Autodesk Inventor part; units mm, degrees
(part 2 of 2)
  arc A565 (31.0706, -18.1829) -> (31.0657, -18.0745) centre (30.9843, -18.1324) ccw
  arc A566 (31.0657, -18.0745) -> (30.4409, -17.2728) centre (21.5601, -24.8386) ccw
  arc A567 (30.4409, -17.2728) -> (30.3559, -17.1866) centre (29.8098, -17.8105) ccw
  arc A568 (29.7735, -16.6368) -> (30.3559, -17.1866) centre (37.4523, -9.0861) ccw
  arc A569 (29.6902, -16.0485) -> (29.7735, -16.6368) centre (30.1301, -16.2863) ccw
  arc A570 (29.6902, -16.0485) -> (29.7499, -15.9376) centre (0, 0) ccw
  arc A571 (30.2868, -15.683) -> (29.7499, -15.9376) centre (30.1906, -16.1737) ccw
  arc A572 (31.0665, -15.8662) -> (30.2868, -15.683) centre (28.2154, -26.2511) ccw
  arc A573 (31.0665, -15.8662) -> (31.1852, -15.8897) centre (31.2863, -15.0667) ccw
  arc A574 (31.1852, -15.8897) -> (32.1985, -15.9695) centre (32.607, -4.31) ccw
  arc A575 (32.1985, -15.9695) -> (32.2917, -15.9137) centre (32.202, -15.8695) ccw
  arc A576 (32.2917, -15.9137) -> (32.5754, -15.3246) centre (0, 0) ccw
  arc A577 (32.5754, -15.3246) -> (32.5609, -15.217) centre (32.4849, -15.282) ccw
  arc A578 (32.5609, -15.217) -> (31.8667, -14.4745) centre (23.6998, -22.806) ccw
  arc A579 (31.8667, -14.4745) -> (31.7743, -14.3964) centre (31.2863, -15.0667) ccw
  arc A580 (31.145, -13.901) -> (31.7743, -14.3964) centre (38.116, -5.6923) ccw
  arc A581 (31.0092, -13.3225) -> (31.145, -13.901) centre (31.4686, -13.5199) ccw
  arc A582 (31.0092, -13.3225) -> (31.0588, -13.2066) centre (0, 0) ccw
  arc A583 (31.5707, -12.905) -> (31.0588, -13.2066) centre (31.5189, -13.4023) ccw
  arc A584 (32.3637, -13.0175) -> (31.5707, -12.905) centre (30.4549, -23.6163) ccw
  arc A585 (32.3637, -13.0175) -> (32.484, -13.0303) centre (32.5109, -12.2015) ccw
  arc A586 (32.484, -13.0303) -> (33.5004, -13.0189) centre (32.8621, -1.3697) ccw
  arc A587 (33.5004, -13.0189) -> (33.5882, -12.9551) centre (33.4949, -12.9191) ccw
  arc A588 (33.5882, -12.9551) -> (33.8179, -12.3429) centre (0, 0) ccw
  arc A589 (33.8179, -12.3429) -> (33.7938, -12.237) centre (33.724, -12.3086) ccw
  arc A590 (33.7938, -12.237) -> (33.0359, -11.5598) centre (25.6487, -20.5897) ccw
  arc A591 (33.0359, -11.5598) -> (32.9369, -11.4902) centre (32.5109, -12.2015) ccw
  arc A592 (32.2657, -11.0532) -> (32.9369, -11.4902) centre (38.4728, -2.2527) ccw
  arc A593 (32.0786, -10.4892) -> (32.2657, -11.0532) centre (32.5539, -10.6446) ccw
  arc A594 (32.0786, -10.4892) -> (32.1176, -10.3694) centre (0, 0) ccw
  arc A595 (32.6004, -10.0231) -> (32.1176, -10.3694) centre (32.5934, -10.523) ccw
  arc A596 (33.4003, -10.0641) -> (32.6004, -10.0231) centre (32.4493, -20.7912) ccw
  arc A597 (33.4003, -10.0641) -> (33.5213, -10.066) centre (33.4738, -9.2382) ccw
  arc A598 (33.5213, -10.066) -> (34.5325, -9.9636) centre (32.8526, 1.5815) ccw
  arc A599 (34.5325, -9.9636) -> (34.6143, -9.8921) centre (34.5181, -9.8646) ccw
  arc A600 (34.6143, -9.8921) -> (34.7882, -9.2618) centre (0, 0) ccw
  arc A601 (34.7882, -9.2618) -> (34.7547, -9.1585) centre (34.6916, -9.236) ccw
  arc A602 (34.7547, -9.1585) -> (33.9391, -8.5519) centre (27.3911, -18.2077) ccw
  arc A603 (33.9391, -8.5519) -> (33.8343, -8.4915) centre (33.4738, -9.2382) ccw
  arc A604 (33.1266, -8.1164) -> (33.8343, -8.4915) centre (38.5198, 1.205) ccw
  arc A605 (32.8897, -7.5715) -> (33.1266, -8.1164) centre (33.377, -7.6837) ccw
  arc A606 (32.8897, -7.5715) -> (32.9178, -7.4487) centre (0, 0) ccw
  arc A607 (33.3676, -7.0604) -> (32.9178, -7.4487) centre (33.4054, -7.559) ccw
  arc A608 (34.1679, -7.0296) -> (33.3676, -7.0604) centre (34.1823, -17.7988) ccw
  arc A609 (34.1679, -7.0296) -> (34.2886, -7.0206) centre (34.1671, -6.2004) ccw
  arc A610 (34.2886, -7.0206) -> (35.2866, -6.828) centre (32.5786, 4.52) ccw
  arc A611 (35.2866, -6.828) -> (35.3616, -6.7495) centre (35.2634, -6.7307) ccw
  arc A612 (35.3616, -6.7495) -> (35.4784, -6.1061) centre (0, 0) ccw
  arc A613 (35.4784, -6.1061) -> (35.4357, -6.0062) centre (35.3798, -6.0891) ccw
  arc A614 (35.4357, -6.0062) -> (34.5691, -5.4752) centre (28.913, -15.6791) ccw
  arc A615 (34.5691, -5.4752) -> (34.4592, -5.4244) centre (34.1671, -6.2004) ccw
  arc A616 (33.7208, -5.1143) -> (34.4592, -5.4244) centre (38.2567, 4.6531) ccw
  arc A617 (33.436, -4.5928) -> (33.7208, -5.1143) centre (33.9314, -4.6608) ccw
  arc A618 (33.436, -4.5928) -> (33.453, -4.4679) centre (0, 0) ccw
  arc A619 (33.8662, -4.041) -> (33.453, -4.4679) centre (33.9486, -4.5341) ccw
  arc A620 (34.6605, -3.9385) -> (33.8662, -4.041) centre (35.6402, -14.6631) ccw
  arc A621 (34.6605, -3.9385) -> (34.7799, -3.9188) centre (34.5854, -3.1127) ccw
  arc A622 (34.7799, -3.9188) -> (35.7566, -3.6374) centre (32.0423, 7.4222) ccw
  arc A623 (35.7566, -3.6374) -> (35.8243, -3.5525) centre (35.7248, -3.5426) ccw
  arc A624 (35.8243, -3.5525) -> (35.8829, -2.9013) centre (0, 0) ccw
  arc A625 (35.8829, -2.9013) -> (35.8315, -2.8056) centre (35.7832, -2.8932) ccw
  arc A626 (35.8315, -2.8056) -> (34.9207, -2.3544) centre (30.202, -13.0242) ccw
  arc A627 (34.9207, -2.3544) -> (34.8068, -2.3137) centre (34.5854, -3.1127) ccw
  arc A628 (34.0435, -2.071) -> (34.8068, -2.3137) centre (37.6856, 8.0636) ccw
  arc A629 (33.7131, -1.5771) -> (34.0435, -2.071) centre (34.2126, -1.6005) ccw
  arc A630 (33.7131, -1.5771) -> (33.7188, -1.4513) centre (0, 0) ccw
  arc A631 (34.0921, -0.989) -> (33.7188, -1.4513) centre (34.2183, -1.4728) ccw
  arc A632 (34.874, -0.8157) -> (34.0921, -0.989) centre (36.8111, -11.4093) ccw
  arc A633 (34.874, -0.8157) -> (34.9912, -0.7853) centre (34.7251, 0) ccw
  arc A634 (34.9912, -0.7853) -> (35.9387, -0.4176) centre (31.2479, 10.2645) ccw
  arc A635 (35.9387, -0.4176) -> (35.9985, -0.3269) centre (35.8985, -0.326) ccw
  arc A636 (35.9985, -0.3269) -> (35.9985, 0.3269) centre (0, 0) ccw
  arc A637 (35.9985, 0.3269) -> (35.9387, 0.4176) centre (35.8985, 0.326) ccw
  arc A638 (35.9387, 0.4176) -> (34.9912, 0.7853) centre (31.2479, -10.2645) ccw
  arc A639 (34.9912, 0.7853) -> (34.874, 0.8157) centre (34.7251, 0) ccw
  arc A640 (34.0921, 0.989) -> (34.874, 0.8157) centre (36.8111, 11.4093) ccw
  arc A641 (33.7188, 1.4513) -> (34.0921, 0.989) centre (34.2183, 1.4728) ccw
  arc A642 (33.7188, 1.4513) -> (33.7131, 1.5771) centre (0, 0) ccw
  arc A643 (34.0435, 2.071) -> (33.7131, 1.5771) centre (34.2126, 1.6005) ccw
  arc A644 (34.8068, 2.3137) -> (34.0435, 2.071) centre (37.6856, -8.0636) ccw
  arc A645 (34.8068, 2.3137) -> (34.9207, 2.3544) centre (34.5854, 3.1127) ccw
  arc A646 (34.9207, 2.3544) -> (35.8315, 2.8056) centre (30.202, 13.0242) ccw
  arc A647 (35.8315, 2.8056) -> (35.8829, 2.9013) centre (35.7832, 2.8932) ccw
  arc A648 (35.8829, 2.9013) -> (35.8243, 3.5525) centre (0, 0) ccw
  arc A649 (35.8243, 3.5525) -> (35.7566, 3.6374) centre (35.7248, 3.5426) ccw
  arc A650 (35.7566, 3.6374) -> (34.7799, 3.9188) centre (32.0423, -7.4222) ccw
  arc A651 (34.7799, 3.9188) -> (34.6605, 3.9385) centre (34.5854, 3.1127) ccw
  arc A652 (33.8662, 4.041) -> (34.6605, 3.9385) centre (35.6402, 14.6631) ccw
  arc A653 (33.453, 4.4679) -> (33.8662, 4.041) centre (33.9486, 4.5341) ccw
  arc A654 (33.453, 4.4679) -> (33.436, 4.5928) centre (0, 0) ccw
  arc A655 (33.7208, 5.1143) -> (33.436, 4.5928) centre (33.9314, 4.6608) ccw
  arc A656 (34.4592, 5.4244) -> (33.7208, 5.1143) centre (38.2567, -4.6531) ccw
  arc A657 (34.4592, 5.4244) -> (34.5691, 5.4752) centre (34.1671, 6.2004) ccw
  arc A658 (34.5691, 5.4752) -> (35.4357, 6.0062) centre (28.913, 15.6791) ccw
  arc A659 (35.4357, 6.0062) -> (35.4784, 6.1061) centre (35.3798, 6.0891) ccw
  arc A660 (35.4784, 6.1061) -> (35.3616, 6.7495) centre (0, 0) ccw
  arc A661 (35.3616, 6.7495) -> (35.2866, 6.828) centre (35.2634, 6.7307) ccw
  arc A662 (35.2866, 6.828) -> (34.2886, 7.0206) centre (32.5786, -4.52) ccw
  arc A663 (34.2886, 7.0206) -> (34.1679, 7.0296) centre (34.1671, 6.2004) ccw
  arc A664 (33.3676, 7.0604) -> (34.1679, 7.0296) centre (34.1823, 17.7988) ccw
  arc A665 (32.9178, 7.4487) -> (33.3676, 7.0604) centre (33.4054, 7.559) ccw
  arc A666 (32.9178, 7.4487) -> (32.8897, 7.5715) centre (0, 0) ccw
  arc A667 (33.1266, 8.1164) -> (32.8897, 7.5715) centre (33.377, 7.6837) ccw
  arc A668 (33.8343, 8.4915) -> (33.1266, 8.1164) centre (38.5198, -1.205) ccw
  arc A669 (33.8343, 8.4915) -> (33.9391, 8.5519) centre (33.4738, 9.2382) ccw
  arc A670 (33.9391, 8.5519) -> (34.7547, 9.1585) centre (27.3911, 18.2077) ccw
  arc A671 (34.7547, 9.1585) -> (34.7882, 9.2618) centre (34.6916, 9.236) ccw
  arc A672 (34.7882, 9.2618) -> (34.6143, 9.8921) centre (0, 0) ccw
  arc A673 (34.6143, 9.8921) -> (34.5325, 9.9636) centre (34.5181, 9.8646) ccw
  arc A674 (34.5325, 9.9636) -> (33.5213, 10.066) centre (32.8526, -1.5815) ccw
  arc A675 (33.5213, 10.066) -> (33.4003, 10.0641) centre (33.4738, 9.2382) ccw
  arc A676 (32.6004, 10.0231) -> (33.4003, 10.0641) centre (32.4493, 20.7912) ccw
  arc A677 (32.1176, 10.3694) -> (32.6004, 10.0231) centre (32.5934, 10.523) ccw
  arc A678 (32.1176, 10.3694) -> (32.0786, 10.4892) centre (0, 0) ccw
  arc A679 (32.2657, 11.0532) -> (32.0786, 10.4892) centre (32.5539, 10.6446) ccw
  arc A680 (32.9369, 11.4902) -> (32.2657, 11.0532) centre (38.4728, 2.2527) ccw
  arc A681 (32.9369, 11.4902) -> (33.0359, 11.5598) centre (32.5109, 12.2015) ccw
  arc A682 (33.0359, 11.5598) -> (33.7938, 12.237) centre (25.6487, 20.5897) ccw
  arc A683 (33.7938, 12.237) -> (33.8179, 12.3429) centre (33.724, 12.3086) ccw
  arc A684 (33.8179, 12.3429) -> (33.5882, 12.9551) centre (0, 0) ccw
  arc A685 (33.5882, 12.9551) -> (33.5004, 13.0189) centre (33.4949, 12.9191) ccw
  arc A686 (33.5004, 13.0189) -> (32.484, 13.0303) centre (32.8621, 1.3697) ccw
  arc A687 (32.484, 13.0303) -> (32.3637, 13.0175) centre (32.5109, 12.2015) ccw
  arc A688 (31.5707, 12.905) -> (32.3637, 13.0175) centre (30.4549, 23.6163) ccw
  arc A689 (31.0588, 13.2066) -> (31.5707, 12.905) centre (31.5189, 13.4023) ccw
  arc A690 (31.0588, 13.2066) -> (31.0092, 13.3225) centre (0, 0) ccw
  arc A691 (31.145, 13.901) -> (31.0092, 13.3225) centre (31.4686, 13.5199) ccw
  arc A692 (31.7743, 14.3964) -> (31.145, 13.901) centre (38.116, 5.6923) ccw
  arc A693 (31.7743, 14.3964) -> (31.8667, 14.4745) centre (31.2863, 15.0667) ccw
  arc A694 (31.8667, 14.4745) -> (32.5609, 15.217) centre (23.6998, 22.806) ccw
  arc A695 (32.5609, 15.217) -> (32.5754, 15.3246) centre (32.4849, 15.282) ccw
  arc A696 (32.5754, 15.3246) -> (32.2917, 15.9137) centre (0, 0) ccw
  arc A697 (32.2917, 15.9137) -> (32.1985, 15.9695) centre (32.202, 15.8695) ccw
  arc A698 (32.1985, 15.9695) -> (31.1852, 15.8897) centre (32.607, 4.31) ccw
  arc A699 (31.1852, 15.8897) -> (31.0665, 15.8662) centre (31.2863, 15.0667) ccw
  arc A700 (30.2868, 15.683) -> (31.0665, 15.8662) centre (28.2154, 26.2511) ccw
  arc A701 (29.7499, 15.9376) -> (30.2868, 15.683) centre (30.1906, 16.1737) ccw
  arc A702 (29.7499, 15.9376) -> (29.6902, 16.0485) centre (0, 0) ccw
  arc A703 (29.7735, 16.6368) -> (29.6902, 16.0485) centre (30.1301, 16.2863) ccw
  arc A704 (30.3559, 17.1866) -> (29.7735, 16.6368) centre (37.4523, 9.0861) ccw
  arc A705 (30.3559, 17.1866) -> (30.4409, 17.2728) centre (29.8098, 17.8105) ccw
  arc A706 (30.4409, 17.2728) -> (31.0657, 18.0745) centre (21.5601, 24.8386) ccw
  arc A707 (31.0657, 18.0745) -> (31.0706, 18.1829) centre (30.9843, 18.1324) ccw
  arc A708 (31.0706, 18.1829) -> (30.7352, 18.7443) centre (0, 0) ccw
  arc A709 (30.7352, 18.7443) -> (30.6374, 18.7914) centre (30.6498, 18.6922) ccw
  arc A710 (30.6374, 18.7914) -> (29.6353, 18.6211) centre (32.0894, 7.2155) ccw
  arc A711 (29.6353, 18.6211) -> (29.5192, 18.5871) centre (29.8098, 17.8105) ccw
  arc A712 (28.7591, 18.3348) -> (29.5192, 18.5871) centre (25.7486, 28.6747) ccw
  arc A713 (28.2015, 18.5402) -> (28.7591, 18.3348) centre (28.6193, 18.8148) ccw
  arc A714 (28.2015, 18.5402) -> (28.1321, 18.6453) centre (0, 0) ccw
  arc A715 (28.1624, 19.2387) -> (28.1321, 18.6453) centre (28.5489, 18.9215) ccw
  arc A716 (28.6931, 19.8385) -> (28.1624, 19.2387) centre (36.487, 12.4067) ccw
  arc A717 (28.6931, 19.8385) -> (28.7701, 19.932) centre (28.0932, 20.4109) ccw
  arc A718 (28.7701, 19.932) -> (29.3205, 20.7864) centre (19.2468, 26.6713) ccw
  arc A719 (29.3205, 20.7864) -> (29.3156, 20.8949) centre (29.2342, 20.8368) ccw
  arc A720 (29.3156, 20.8949) -> (28.9312, 21.4239) centre (0, 0) ccw
  arc A721 (28.9312, 21.4239) -> (28.8296, 21.4621) centre (28.8509, 21.3644) ccw
  arc A722 (28.8296, 21.4621) -> (27.8469, 21.2027) centre (31.3135, 10.0629) ccw
  arc A723 (27.8469, 21.2027) -> (27.7342, 21.1584) centre (28.0932, 20.4109) ccw
  arc A724 (26.9998, 20.8389) -> (27.7342, 21.1584) centre (23.0746, 30.8673) ccw
  arc A725 (26.426, 20.9935) -> (26.9998, 20.8389) centre (26.8175, 21.3045) ccw
  arc A726 (26.426, 20.9935) -> (26.3475, 21.092) centre (0, 0) ccw
  arc A727 (26.3244, 21.6857) -> (26.3475, 21.092) centre (26.7378, 21.4045) ccw
  arc A728 (26.7993, 22.3307) -> (26.3244, 21.6857) centre (35.228, 15.6275) ccw
  arc A729 (26.7993, 22.3307) -> (26.8676, 22.4306) centre (26.1505, 22.847) ccw
  arc A730 (26.8676, 22.4306) -> (27.3392, 23.331) centre (16.7785, 28.2892) ccw
  arc A731 (27.3392, 23.331) -> (27.3246, 23.4386) centre (27.2487, 23.3735) ccw
  arc A732 (27.3246, 23.4386) -> (26.8943, 23.931) centre (0, 0) ccw
  arc A733 (26.8943, 23.931) -> (26.7897, 23.96) centre (26.8196, 23.8646) ccw
  arc A734 (26.7897, 23.96) -> (25.8342, 23.6135) centre (30.2854, 12.8293) ccw
  arc A735 (25.8342, 23.6135) -> (25.726, 23.5592) centre (26.1505, 22.847) ccw
  arc A736 (25.0231, 23.1753) -> (25.726, 23.5592) centre (20.2148, 32.8115) ccw
  arc A737 (24.4378, 23.2778) -> (25.0231, 23.1753) centre (24.7999, 23.6226) ccw
  arc A738 (24.4378, 23.2778) -> (24.3508, 23.3689) centre (0, 0) ccw
  arc A739 (24.2746, 23.9582) -> (24.3508, 23.3689) centre (24.7115, 23.7151) ccw
  arc A740 (24.6897, 24.6431) -> (24.2746, 23.9582) centre (33.6854, 18.7224) ccw
  arc A741 (24.6897, 24.6431) -> (24.7487, 24.7487) centre (23.9973, 25.0992) ccw
  arc A742 (24.7487, 24.7487) -> (25.1378, 25.6877) centre (14.1751, 29.6793) ccw
  arc A743 (25.1378, 25.6877) -> (25.1135, 25.7936) centre (25.0438, 25.722) ccw
  arc A744 (25.1135, 25.7936) -> (24.6409, 26.2455) centre (0, 0) ccw
  arc A745 (24.6409, 26.2455) -> (24.5341, 26.2649) centre (24.5725, 26.1726) ccw
  arc A746 (24.5341, 26.2649) -> (23.6135, 25.8342) centre (29.0134, 15.4924) ccw
  arc A747 (23.6135, 25.8342) -> (23.5106, 25.7705) centre (23.9973, 25.0992) ccw
  arc A748 (22.845, 25.325) -> (23.5106, 25.7705) centre (17.1922, 34.4914) ccw
  arc A749 (22.2528, 25.3747) -> (22.845, 25.325) centre (22.5825, 25.7506) ccw
  arc A750 (22.2528, 25.3747) -> (22.158, 25.4576) centre (0, 0) ccw
  arc A751 (22.0293, 26.0377) -> (22.158, 25.4576) centre (22.4862, 25.8347) ccw
  arc A752 (22.3813, 26.757) -> (22.0293, 26.0377) centre (31.8715, 21.6665) ccw
  arc A753 (22.3813, 26.757) -> (22.4306, 26.8676) centre (21.6508, 27.1492) ccw
  arc A754 (22.4306, 26.8676) -> (22.7339, 27.8377) centre (11.4577, 30.8305) ccw
  arc A755 (22.7339, 27.8377) -> (22.7003, 27.9409) centre (22.6373, 27.8633) ccw
  arc A756 (22.7003, 27.9409) -> (22.1891, 28.3486) centre (0, 0) ccw
  arc A757 (22.1891, 28.3486) -> (22.0809, 28.3584) centre (22.1275, 28.2699) ccw
  arc A758 (22.0809, 28.3584) -> (21.2027, 27.8469) centre (27.5079, 18.0308) ccw
  arc A759 (21.2027, 27.8469) -> (21.1059, 27.7742) centre (21.6508, 27.1492) ccw
  arc A760 (20.4829, 27.2709) -> (21.1059, 27.7742) centre (14.0312, 35.8937) ccw
  arc A761 (19.8887, 27.2672) -> (20.4829, 27.2709) centre (20.1833, 27.6712) ccw
  arc A762 (19.8887, 27.2672) -> (19.7868, 27.3413) centre (0, 0) ccw
  arc A763 (19.6066, 27.9075) -> (19.7868, 27.3413) centre (20.0799, 27.7464) ccw
  arc A764 (19.8928, 28.6556) -> (19.6066, 27.9075) centre (29.801, 24.4362) ccw
  arc A765 (19.8928, 28.6556) -> (19.932, 28.7701) centre (19.13, 28.9807) ccw
  arc A766 (19.932, 28.7701) -> (20.1471, 29.7634) centre (8.6479, 31.7334) ccw
  arc A767 (20.1471, 29.7634) -> (20.1043, 29.8633) centre (20.0485, 29.7803) ccw
  arc A768 (20.1043, 29.8633) -> (19.5586, 30.2235) centre (0, 0) ccw
  arc A769 (19.5586, 30.2235) -> (19.45, 30.2236) centre (19.5043, 30.1396) ccw
  arc A770 (19.45, 30.2236) -> (18.6211, 29.6353) centre (25.7809, 20.424) ccw
  arc A771 (18.6211, 29.6353) -> (18.5312, 29.5543) centre (19.13, 28.9807) ccw
  arc A772 (17.9559, 28.9971) -> (18.5312, 29.5543) centre (10.7572, 37.0069) ccw
  arc A773 (17.3644, 28.9403) -> (17.9559, 28.9971) centre (17.6216, 29.369) ccw
  arc A774 (17.3644, 28.9403) -> (17.2562, 29.0049) centre (0, 0) ccw
  arc A775 (17.026, 29.5527) -> (17.2562, 29.0049) centre (17.5119, 29.4346) ccw
  arc A776 (17.244, 30.3234) -> (17.026, 29.5527) centre (27.4906, 27.0092) ccw
  arc A777 (17.244, 30.3234) -> (17.2728, 30.4409) centre (16.4552, 30.5788) ccw
  arc A778 (17.2728, 30.4409) -> (17.398, 31.4496) centre (5.7685, 32.3808) ccw
  arc A779 (17.398, 31.4496) -> (17.3465, 31.5452) centre (17.2983, 31.4576) ccw
  arc A780 (17.3465, 31.5452) -> (16.7707, 31.8551) centre (0, 0) ccw
  arc A781 (16.7707, 31.8551) -> (16.6625, 31.8454) centre (16.7241, 31.7666) ccw
  arc A782 (16.6625, 31.8454) -> (15.8897, 31.1852) centre (23.8463, 22.6528) ccw
  arc A783 (15.8897, 31.1852) -> (15.8074, 31.0964) centre (16.4552, 30.5788) ccw
  arc A784 (15.2843, 30.49) -> (15.8074, 31.0964) centre (7.3967, 37.8222) ccw
  arc A785 (14.7003, 30.3803) -> (15.2843, 30.49) centre (14.9181, 30.8304) ccw
  arc A786 (14.7003, 30.3803) -> (14.5868, 30.435) centre (0, 0) ccw
  arc A787 (14.3084, 30.9599) -> (14.5868, 30.435) centre (14.8029, 30.8859) ccw
  arc A788 (14.4564, 31.747) -> (14.3084, 30.9599) centre (24.9588, 29.3647) ccw
  arc A789 (14.4564, 31.747) -> (14.4745, 31.8667) centre (13.6479, 31.9307) ccw
  arc A790 (14.4745, 31.8667) -> (14.5088, 32.8825) centre (2.8427, 32.7676) ccw
  arc A791 (14.5088, 32.8825) -> (14.449, 32.9731) centre (14.4088, 32.8815) ccw
  arc A792 (14.449, 32.9731) -> (13.8477, 33.2301) centre (0, 0) ccw
  arc A793 (13.8477, 33.2301) -> (13.7408, 33.2108) centre (13.8092, 33.1378) ccw
  arc A794 (13.7408, 33.2108) -> (13.0303, 32.484) centre (21.7197, 24.6991) ccw
  arc A795 (13.0303, 32.484) -> (12.9563, 32.3882) centre (13.6479, 31.9307) ccw
  arc A796 (12.4897, 31.7373) -> (12.9563, 32.3882) centre (3.9765, 38.333) ccw
  arc A797 (11.9179, 31.5757) -> (12.4897, 31.7373) centre (12.0944, 32.0435) ccw
  arc A798 (11.9179, 31.5757) -> (11.7999, 31.62) centre (0, 0) ccw
  arc A799 (11.4756, 32.1179) -> (11.7999, 31.62) centre (11.9747, 32.0885) ccw
  arc A800 (11.5524, 32.9151) -> (11.4756, 32.1179) centre (22.2261, 31.4838) ccw
  arc A801 (11.5524, 32.9151) -> (11.5598, 33.0359) centre (10.7307, 33.0256) ccw
  arc A802 (11.5598, 33.0359) -> (11.5028, 34.0507) centre (-0.106, 32.8905) ccw
  arc A803 (11.5028, 34.0507) -> (11.4351, 34.1356) centre (11.4033, 34.0408) ccw
  arc A804 (11.4351, 34.1356) -> (10.8132, 34.3377) centre (0, 0) ccw
  arc A805 (10.8132, 34.3377) -> (10.7085, 34.3088) centre (10.7832, 34.2423) ccw
  arc A806 (10.7085, 34.3088) -> (10.066, 33.5213) centre (19.4183, 26.5467) ccw
  arc A807 (10.066, 33.5213) -> (10.0009, 33.4192) centre (10.7307, 33.0256) ccw
  arc A808 (9.5945, 32.7291) -> (10.0009, 33.4192) centre (0.5244, 38.5351) ccw
  arc A809 (9.0395, 32.5169) -> (9.5945, 32.7291) centre (9.1734, 32.9987) ccw
  arc A810 (9.0395, 32.5169) -> (8.918, 32.5504) centre (0, 0) ccw
  arc A811 (8.5504, 33.0173) -> (8.918, 32.5504) centre (9.0501, 33.0327) ccw
  arc A812 (8.5554, 33.8182) -> (8.5504, 33.0173) centre (19.3145, 33.3494) ccw
  arc A813 (8.5554, 33.8182) -> (8.5519, 33.9391) centre (7.7271, 33.8545) ccw
  arc A814 (8.5519, 33.9391) -> (8.4042, 34.9447) centre (-3.0538, 32.7486) ccw
  arc A815 (8.4042, 34.9447) -> (8.3292, 35.0232) centre (8.306, 34.9259) ccw
  arc A816 (8.3292, 35.0232) -> (7.6917, 35.1687) centre (0, 0) ccw
  arc A817 (7.6917, 35.1687) -> (7.59, 35.1306) centre (7.6703, 35.071) ccw
  arc A818 (7.59, 35.1306) -> (7.0206, 34.2886) centre (16.9605, 28.1804) ccw
  arc A819 (7.0206, 34.2886) -> (6.965, 34.1812) centre (7.7271, 33.8545) ccw
  arc A820 (6.622, 33.4574) -> (6.965, 34.1812) centre (-2.932, 38.427) ccw
  arc A821 (6.0883, 33.1963) -> (6.622, 33.4574) centre (6.1785, 33.6881) ccw
  arc A822 (6.0883, 33.1963) -> (5.9643, 33.2188) centre (0, 0) ccw
  arc A823 (5.5563, 33.6508) -> (5.9643, 33.2188) centre (6.0527, 33.7109) ccw
  arc A824 (5.4896, 34.4489) -> (5.5563, 33.6508) centre (16.2473, 34.9465) ccw
  arc A825 (5.4896, 34.4489) -> (5.4752, 34.5691) centre (4.6613, 34.4109) ccw
  arc A826 (5.4752, 34.5691) -> (5.238, 35.5574) centre (-5.9771, 32.343) ccw
  arc A827 (5.238, 35.5574) -> (5.1562, 35.6288) centre (5.1419, 35.5299) ccw
  arc A828 (5.1562, 35.6288) -> (4.5082, 35.7166) centre (0, 0) ccw
  arc A829 (4.5082, 35.7166) -> (4.4104, 35.6695) centre (4.4957, 35.6174) ccw
  arc A830 (4.4104, 35.6695) -> (3.9188, 34.7799) centre (14.3661, 29.5873) ccw
  arc A831 (3.9188, 34.7799) -> (3.8729, 34.6679) centre (4.6613, 34.4109) ccw
  arc A832 (3.5963, 33.9163) -> (3.8729, 34.6679) centre (-6.3647, 38.0095) ccw
  arc A833 (3.0881, 33.6084) -> (3.5963, 33.9163) centre (3.1338, 34.1063) ccw
  arc A834 (3.0881, 33.6084) -> (2.9626, 33.6197) centre (0, 0) ccw
  arc A835 (2.5175, 34.0134) -> (2.9626, 33.6197) centre (3.0065, 34.1178) ccw
  arc A836 (2.3795, 34.8023) -> (2.5175, 34.0134) centre (13.0493, 36.2622) ccw
  arc A837 (2.3795, 34.8023) -> (2.3544, 34.9207) centre (1.5579, 34.6902) ccw
  arc A838 (2.3544, 34.9207) -> (2.0296, 35.8838) centre (-8.8523, 31.677) ccw
  arc A839 (2.0296, 35.8838) -> (1.9417, 35.9476) centre (1.9363, 35.8477) ccw
  arc A840 (1.9417, 35.9476) -> (1.2884, 35.9769) centre (0, 0) ccw
  constraints: 1680 point on circle, 841 centre point
extrude "Extrusion1" cut sketch "Sketch_2" against normal blind 10
ref_plane "teeth_to_body_XY" through (0, 0, 0) normal (1, 0, 0) x (0, 0, -1)
ref_plane "teeth_to_body_YZ" through (0, 0, 0) normal (0, 0, -1) x (0, 1, 0)
ref_plane "teeth_to_body_ZX" through (0, 0, 0) normal (0, 1, 0) x (1, 0, 0)
body "Solid1"
